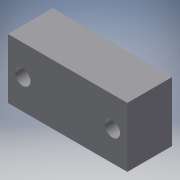
# Autodesk Inventor part: IC end caps
Saved by Autodesk Inventor 2018 (Build 220112000, 112)
## iProperties
Created: 2018-02-03
Part Number: IC end caps
Material: Generic
Document SubType Name: Modeling
Designer: Luke
Density: 1 g/cm^3
Appearance: Default
Author: Luke
Autodesk Inventor part; units mm, degrees
ref_plane "YZ Plane" through (0, 0, 0) normal (1, 0, 0) x (0, 1, 0)
ref_plane "XZ Plane" through (0, 0, 0) normal (0, 1, 0) x (-1, 0, 0)
ref_plane "XY Plane" through (0, 0, 0) normal (0, 0, 1) x (1, 0, 0)
sketch "Sketch1" plane through (0, 0, 0) normal (0, 0, 1) x (1, 0, 0)
  line L0 (0, 0) -> (-101.6, 0)
  line L1 (-101.6, 0) -> (-101.6, -50.8)
  line L2 (-101.6, -50.8) -> (0, -50.8)
  line L3 (0, -50.8) -> (0, 0)
  circle A0 centre (-88.9, -25.4) radius 6.477
  circle A1 centre (-12.7, -25.4) radius 6.477
  dimension "d0" = 101.6
  dimension "d1" = 50.8
  dimension "d2" = 12.954
  dimension "d3" = 12.954
  dimension "d4" = 12.7
  dimension "d5" = 12.7
  dimension "d6" = 25.4
  dimension "d7" = 25.4
  constraints: 8 end point, 2 centre point, 2 parallel, 1 horizontal, 1 perpendicular
  measures "d0" distance of L2.end L1.end
  measures "d1" distance of L1.end L0.end
  measures "d2" diameter of A0
  measures "d3" diameter of A1
  measures "d4" distance from line of L1 A0.centre
  measures "d5" distance from line of L3 A1.centre
  measures "d6" distance from line of L0 A1.centre
  measures "d7" distance from line of L0 A0.centre
extrude "Extrusion1" add sketch "Sketch1" along normal blind 12.7
body "Solid1"
